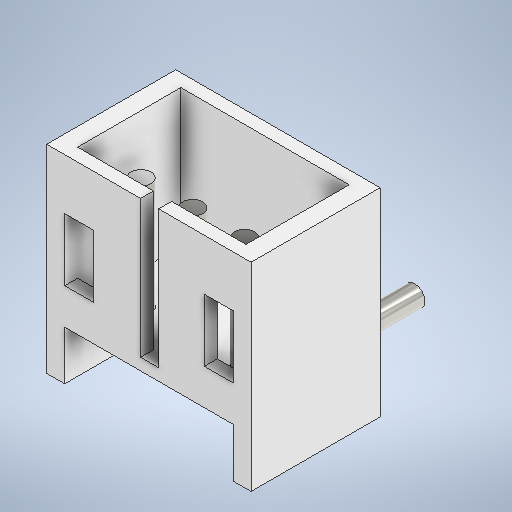
# Autodesk Inventor part: 2SH-C-03-TR
Saved by Autodesk Inventor 2025 (Build 290162000, 162)
## iProperties
Company: The University of Winnipeg
Created: 2026-07-15
Part Number: 2SH-C-03-TR
Material: Generic
Catalog Web Link: https://www.digikey.ca/en/products/detail/adam-tech/2SH-C-03-TR/9830368
Description: CONN HEADER R/A 3POS 2MM
Vendor: Digikey
Document SubType Name: Modeling
Designer: Tapendra BC
Density: 1 g/cm^3
Appearance: Default
Author: Tapendra BC
Autodesk Inventor part; units mm, degrees
ref_plane "YZ Plane" through (0, 0, 0) normal (1, 0, 0) x (0, 1, 0)
ref_plane "XZ Plane" through (0, 0, 0) normal (0, 1, 0) x (-1, 0, 0)
ref_plane "XY Plane" through (0, 0, 0) normal (0, 0, 1) x (1, 0, 0)
sketch "Sketch1" plane through (0, 0, 0) normal (0, 0, 1) x (1, 0, 0)
  line L0 (-3.9624, 3.8481) -> (3.9624, 3.8481)
  line L1 (3.9624, 3.8481) -> (3.9624, -3.8481)
  line L2 (3.9624, -3.8481) -> (-3.9624, -3.8481)
  line L3 (-3.9624, -3.8481) -> (-3.9624, 3.8481)
  line L4 (-3.9624, 3.8481) -> (3.9624, -3.8481) construction
  line L5 (3.9624, 3.8481) -> (-3.9624, -3.8481) construction
  point P0 (0, 0)
  dimension "d0" = 7.6962
  dimension "d1" = 7.9248
  constraints: 12 end point, 2 midpoint, 2 parallel, 1 horizontal, 1 perpendicular
  measures "d0" distance of L0.end L1.end
  measures "d1" distance of L1.end L2.end
extrude "Extrusion1" add sketch "Sketch1" along normal blind 5.0038
sketch "Sketch4" plane through (-3.9624, 3.8481, 0) normal (0, 1, 0) x (1, 0, 0)
  line L0 (7.2277, -4.5029) -> (0.6971, -4.5029)
  line L1 (0.6971, -4.5029) -> (0.6971, -0.5009)
  line L2 (0.6971, -0.5009) -> (7.2277, -0.5009)
  line L3 (7.2277, -0.5009) -> (7.2277, -4.5029)
  line L4 (7.2277, -4.5029) -> (0.6971, -0.5009) construction
  line L5 (0.6971, -4.5029) -> (7.2277, -0.5009) construction
  line L6 (7.9248, -5.0038) -> (0, -5.0038) projected
  point P0 (3.9624, 0)
  point P1 (3.9624, -2.5019)
  dimension "d16" = 2.5019
  constraints: 12 end point, 2 midpoint, 2 parallel, 1 horizontal, 1 perpendicular
  measures "d16" distance from line of L6 point (3.962, -2.502)
extrude "Extrusion3" cut sketch "Sketch4" against normal blind 5.334
sketch "Sketch5" plane through (-3.9624, -3.8481, 0) normal (0, -1, 0) x (1, 0, 0)
  line L0 (7.9248, 5.0038) -> (0, 5.0038) projected
  line L1 (7.9248, 0) -> (0, 0) projected
  line L2 (0.6971, 5.0038) -> (7.2277, 5.0038)
  line L3 (7.2277, 5.0038) -> (7.2277, 0)
  line L4 (7.2277, 0) -> (0.6971, 0)
  line L5 (0.6971, 0) -> (0.6971, 5.0038)
  point P0 (3.9624, 0)
  point P1 (0.6971, 4.5029)
  point P2 (7.2277, 0.5009)
  constraints: 8 end point, 2 parallel, 2 point on line, 1 horizontal, 1 perpendicular
extrude "Extrusion4" cut sketch "Sketch5" against normal blind 1.905
sketch "Sketch9" plane through (0, 0, 5.0038) normal (0, 0, 1) x (1, 0, 0)
  line L0 (3.2653, 3.8481) -> (-3.2653, 3.8481) projected
  line L1 (-3.2653, -1.4859) -> (3.2653, -1.4859) projected
  line L2 (0.3773, 3.8481) -> (-0.3246, 3.8481)
  line L3 (-0.3246, 3.8481) -> (-0.3246, -1.4859)
  line L4 (-0.3246, -1.4859) -> (0.3773, -1.4859)
  line L5 (0.3773, -1.4859) -> (0.3773, 3.8481)
  line L6 (3.2653, 3.8481) -> (3.2653, -1.4859) projected
  line L7 (3.2653, -0.5528) -> (2.1497, -0.5528)
  line L8 (2.1497, -0.5528) -> (2.1497, 1.8689)
  line L9 (2.1497, 1.8689) -> (3.2653, 1.8689)
  line L10 (3.2653, 1.8689) -> (3.2653, -0.5528)
  line L11 (-3.2653, 3.8481) -> (-3.2653, -1.4859) projected
  line L12 (-3.2653, -0.5528) -> (-2.1497, -0.5528)
  line L13 (-2.1497, -0.5528) -> (-2.1497, 1.8689)
  line L14 (-2.1497, 1.8689) -> (-3.2653, 1.8689)
  line L15 (-3.2653, 1.8689) -> (-3.2653, -0.5528)
  point P0 (0, 0)
  dimension "d36" = 1.1156
  dimension "d37" = 1.1156
  constraints: 24 end point, 6 parallel, 6 point on line, 3 horizontal, 3 perpendicular
  measures "d36" distance between parallel lines of L15 L13
  measures "d37" distance between parallel lines of L6 L8
extrude "Extrusion7" cut sketch "Sketch9" against normal up to surface (0.5009 mm away) contours L5 L1 L3 L0 | L6 L7 L8 L9 | L14 L13 L12 L11
sketch "Sketch10" plane through (-3.9624, -1.4859, 0) normal (0, 1, 0) x (1, 0, 0)
  circle A0 centre (3.961, -3.302) radius 0.3937
  line L0 (7.9248, -5.0038) -> (4.3397, -5.0038) projected
  line L1 (0.6971, -4.5029) -> (0.6971, -0.5009) projected
  circle A1 centre (1.9544, -3.302) radius 0.3937
  line L2 (3.6378, -5.0038) -> (0, -5.0038) projected
  circle A2 centre (5.9676, -3.302) radius 0.3937
  point P0 (3.9624, 0)
  dimension "d40" = 1.7018
  dimension "d41" = 0.7874
  dimension "d42" = 3.2639
  dimension "d43" = 0.7874
  dimension "d44" = 1.7018
  dimension "d45" = 2.0066
  dimension "d46" = 0.7874
  dimension "d47" = 1.7018
  dimension "d48" = 2.0066
  constraints: 3 centre point
  measures "d40" distance from line of L0 A0.centre
  measures "d41" diameter of A0
  measures "d42" distance from line of L1 A0.centre
  measures "d43" diameter of A1
  measures "d44" distance from line of L2 A1.centre
  measures "d45" distance of A1.centre A0.centre
  measures "d46" diameter of A2
  measures "d47" distance from line of L0 A2.centre
  measures "d48" distance of A0.centre A2.centre
ref_plane "Work Plane1" through (-0.0014, -1.4859, 3.302) normal (-1, 0, 0) x (0, 0, 1)
sketch "Sketch11" plane through (-0.0014, -1.4859, 3.302) normal (-1, 0, 0) x (0, 0, 1)
  line L0 (-2.8011, 0) -> (1.2009, 0) projected
  line L1 (0.0001, 0) -> (0.0001, 4.334)
  line L2 (-2.8011, 5.334) -> (1.2009, 5.334) projected
  line L3 (-4.4984, -0.9144) -> (-6.604, -0.9144)
  line L4 (-3.302, -2.3622) -> (-3.302, 5.334) projected
  line L5 (-3.302, 5.334) -> (1.7018, 5.334) projected
  line L6 (-3.302, -0.9144) -> (-4.4984, -0.9144)
  line L7 (-3.302, -0.9144) -> (-0.5079, -0.9144)
  line L8 (0.0001, -0.4064) -> (0.0001, 0)
  arc A0 (-0.5079, -0.9144) -> (0.0001, -0.4064) centre (-0.5079, -0.4064) ccw
  point P0 (-3.302, 1.4859)
  dimension "d49" = 1
  dimension "d50" = 3.302
  dimension "d51" = 6.2484
  dimension "d52" = 0.508
  constraints: 10 end point, 2 perpendicular, 2 point on circle, 2 point on line, 2 tangent, 1 centre point, 1 horizontal
  measures "d49" distance from line of L2 L1.end
  measures "d50" distance from line of L3.end L4
  measures "d51" distance from line of L5 L3.end
  measures "d52" radius of A0
sweep "Sweep1" add profiles "Sketch10" path "Sketch11" path curves L3 L6 L7 A0 L8 L1
equation "\"d37\" = d36"
equation "\"d44\" = d40"
equation "\"d47\" = d40"
equation "\"d48\" = d45"
body "Solid1"
